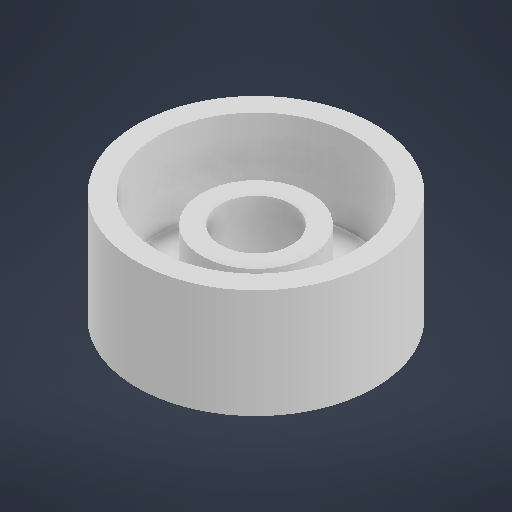
# Autodesk Inventor part: Колесо
Saved by Autodesk Inventor 2026.2 (Build 302298000, 298)
## iProperties
Created: 2026-02-19
Part Number: Колесо
Material: Типовые
Document SubType Name: Modeling
Designer: Leonid
Density: 1 g/cm^3
Appearance: По умолчанию
Author: Leonid
Autodesk Inventor part; units mm, degrees
ref_plane "YZ Plane" through (0, 0, 0) normal (1, 0, 0) x (0, 1, 0)
ref_plane "XZ Plane" through (0, 0, 0) normal (0, 1, 0) x (-1, 0, 0)
ref_plane "XY Plane" through (0, 0, 0) normal (0, 0, 1) x (1, 0, 0)
sketch "Эскиз1" plane through (0, 0, 0) normal (0, 1, 0) x (-1, 0, 0)
  circle A0 centre (0, 0) radius 8.75
  circle A1 centre (0, 0) radius 2.6
  circle A2 centre (0, 0) radius 4
  circle A3 centre (0, 0) radius 7.25
  point P0 (-0.75, 3.9291)
  point P1 (-0.6797, 7.2181)
  point P2 (0.6797, 7.2181)
  point P3 (0.75, 3.9291)
  dimension "d1" = 5.2
  dimension "d2" = 8
  dimension "d41" = 17.5
  dimension "d43" = 1.5
  constraints: 4 centre point, 4 coincident, 4 point on circle
  measures "d1" diameter of A1
  measures "d2" diameter of A2
  measures "d41" diameter of A0
  measures "d43" radial gap between concentric circles of A3 A0
extrude "Выдавливание1" add sketch "Эскиз1" along normal blind 8 contours A0
extrude "Выдавливание7" add sketch "Эскиз1" along normal blind 6 contours A2
extrude "Выдавливание8" add sketch "Эскиз1" along normal blind 1.75 contours A3
